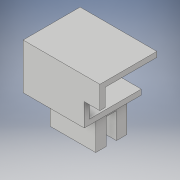
# Autodesk Inventor part: battery-holder-two
Saved by Autodesk Inventor 2019 (Build 230136000, 136)
## iProperties
Created: 2019-05-03
Part Number: battery-holder-two
Material: Generic
Document SubType Name: Modeling
Designer: Tesler
Density: 1 g/cm^3
Appearance: Default
Author: Tesler
## iProperties of the stored document battery-holder-two_3DPrint.ipt
Created: 2019-05-03
Part Number: battery-holder-two_3DPrint
Material: Generic
Document SubType Name: Modeling
Designer: Tesler
Density: 1 g/cm^3
Appearance: Default
Author: Tesler
Autodesk Inventor part; units mm, degrees
ref_plane "YZ Plane" through (0, 0, 0) normal (1, 0, 0) x (0, 1, 0)
ref_plane "XZ Plane" through (0, 0, 0) normal (0, 1, 0) x (-1, 0, 0)
ref_plane "XY Plane" through (0, 0, 0) normal (0, 0, 1) x (1, 0, 0)
sketch "Sketch2" plane through (0, -7.5, 2.5) normal (1, 0, 0) x (0, 1, 0)
  line L0 (0, 0) -> (12.5, 0)
  line L1 (12.5, 0) -> (12.5, -5)
  line L2 (12.5, -5) -> (0, -5)
  line L3 (0, 0) -> (0, 5)
  line L4 (0, 5) -> (15, 5)
  line L5 (15, 5) -> (15, -10)
  line L6 (15, -10) -> (0, -10)
  line L7 (0, -10) -> (0, -5)
  dimension "d11" = 12.5
  dimension "d10" = 5
  dimension "d9" = 15
  dimension "d8" = 15
  dimension "d12" = 5
  constraints: 16 end point, 5 perpendicular, 1 horizontal, 1 parallel, 1 point on line, 1 vertical
  measures "d11" distance of L1.end L2.end
  measures "d10" distance of L0.start L3.end
  measures "d9" distance of L3.end L4.end
  measures "d8" distance of L4.end L5.end
  measures "d12" distance of L0.end L1.end
extrude "Extrusion2" add sketch "Sketch2" along normal blind 22
sketch "Sketch4" plane through (0, -7.5, -7.5) normal (0, 0, -1) x (-1, 0, 0)
  line L0 (0, 0) -> (0, 15) projected
  line L1 (0, 15) -> (-22, 15) projected
  line L2 (-22, 0) -> (-22, 15) projected
  line L3 (0, 0) -> (-22, 0) projected
  line L4 (5.5, 15) -> (-31.5, 15)
  line L5 (-31.5, 37) -> (-31.5, 34.5)
  line L6 (5.5, 15) -> (5.5, 37)
  line L7 (5.5, 37) -> (3, 37)
  line L8 (3, 34.5) -> (3, 17.5)
  line L9 (3, 17.5) -> (-31.5, 17.5)
  line L10 (-31.5, 17.5) -> (-31.5, 15)
  line L11 (3, 37) -> (-31.5, 37)
  line L12 (3, 34.5) -> (-31.5, 34.5)
  point P0 (0, 7.5)
  dimension "d29" = 5.5
  dimension "d32" = 19.5
  dimension "d33" = 2.5
  dimension "d34" = 2.5
  dimension "d35" = 22
  dimension "d38" = 15
  dimension "d58" = 2.5
  dimension "d65" = 37
  dimension "d66" = 34.5
  dimension "d67" = 2.5
  constraints: 18 end point, 3 perpendicular, 2 vertical, 1 horizontal, 1 parallel
  measures "d29" distance from line of L0 L4.start
  measures "d32" distance of L5.start L9.end
  measures "d33" distance of L6.end L7.end
  measures "d34" distance between parallel lines of L9 L1
  measures "d35" distance between parallel lines of L7 L4
  measures "d38" distance between parallel lines of L4 L3
  measures "d58" distance between parallel lines of L11 L12
  measures "d65" distance between parallel lines of L6 L5
  measures "d66" distance of L7.end L5.start
  measures "d67" distance between parallel lines of L6 L8
extrude "Extrusion4" add sketch "Sketch4" against normal blind 20 and the other way blind 5 contours L1 L4 L10 L9 L8 L12 L5 L11 L7 L6
sketch "Sketch9" plane through (0, -7.5, 12.5) normal (0, 0, 1) x (1, 0, 0)
  line L0 (-5.5, 37) -> (31.5, 37) projected
  line L1 (-5.5, 37) -> (-5.5, 15) projected
  line L2 (31.5, 37) -> (-5.5, 37)
  line L3 (-5.5, 37) -> (-5.5, 15)
  line L4 (-5.5, 15) -> (31.5, 15)
  line L5 (31.5, 15) -> (31.5, 37)
  point P0 (0, 7.5)
  constraints: 8 end point, 2 parallel, 1 horizontal, 1 perpendicular
extrude "Extrusion9" add sketch "Sketch9" along normal blind 2.5
sketch "Sketch10" plane through (31.5, 7.5, -12.5) normal (1, 0, 0) x (0, 0, -1)
  line L0 (-27.5, 22) -> (-27.5, 0) projected
  line L1 (0, 0) -> (-27.5, 0) projected
  line L2 (-27.5, 11) -> (0, 11)
  line L3 (0, 11) -> (0, 0)
  line L4 (0, 0) -> (-27.5, 0)
  line L5 (-27.5, 0) -> (-27.5, 11)
  point P0 (-12.5, -7.5)
  constraints: 8 end point, 2 parallel, 1 horizontal, 1 midpoint, 1 perpendicular
extrude "Extrusion10" cut sketch "Sketch10" against normal blind 7.5
body "Solid2"
